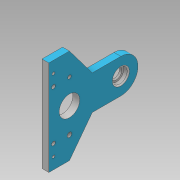
# Autodesk Inventor part: 탑(모터쪽옆면수정)
Saved by Autodesk Inventor 2018 (Build 220112000, 112)
## iProperties
Created: 2018-04-17
Part Number: 탑(모터쪽옆면수정)
Material: 일반
Document SubType Name: Modeling
Designer: CK
Density: 1 g/cm^3
Appearance: 기본값
Mass: 19.8797 g
Surface Area: 92.9275 cm^2
Volume: 19.8797 cm^3
Author: CK
Autodesk Inventor part; units mm, degrees
ref_plane "YZ Plane" through (0, 0, 0) normal (1, 0, 0) x (0, 1, 0)
ref_plane "XZ Plane" through (0, 0, 0) normal (0, 1, 0) x (-1, 0, 0)
ref_plane "XY Plane" through (0, 0, 0) normal (0, 0, 1) x (1, 0, 0)
sketch "스케치1" plane through (0, 0, 0) normal (1, 0, 0) x (0, 1, 0)
  line L0 (0, -41.5) -> (18, -41.5)
  line L1 (18, -41.5) -> (18, 59.6584) construction
  line L2 (0, 0) -> (0, -41.5)
  line L3 (84.3904, 0) -> (-15.1692, 0) construction
  arc A0 (63, -15) -> (78, 0) centre (63, 0) ccw
  line L4 (63, -15) -> (38, -15)
  line L5 (38, -15) -> (18, -41.5)
  line L6 (0, 41.5) -> (18, 41.5)
  line L7 (0, 0) -> (0, 41.5)
  arc A1 (78, 0) -> (63, 15) centre (63, 0) ccw
  line L8 (63, 15) -> (38, 15)
  line L9 (38, 15) -> (18, 41.5)
  dimension "d0" = 18
  dimension "d8" = 45
  dimension "d9" = 25
  constraints: 20 end point, 4 point on circle, 4 symmetric about line, 2 centre point, 2 horizontal, 2 point on line, 2 vertical, 1 other
  measures "d0" distance of L0.start L0.end
  measures "d8" distance from line of L1 A0.centre
  measures "d9" distance of L4.start L4.end
extrude "돌출1" add sketch "스케치1" along normal blind 6
sketch "스케치2" plane through (6, 0, 0) normal (1, 0, 0) x (0, 0, -1)
  line L0 (-58.8675, 4) -> (65.7315, 4) construction
  line L1 (-41.5, 0) -> (41.5, 0) projected
  circle A0 centre (31.5, 4) radius 1.15
  circle A1 centre (21.5, 4) radius 1.65
  line L2 (41.5, 0) -> (41.5, 18) projected
  line L3 (0, 13.8041) -> (0, -7.7982) construction
  circle A2 centre (-31.5, 4) radius 1.15
  circle A3 centre (-21.5, 4) radius 1.65
  point P0 (0, 0)
  dimension "d12" = 4
  dimension "d13" = 2.3
  dimension "d14" = 3.3
  dimension "d15" = 10
  dimension "d16" = 20
  dimension "d32" = 21.5
  constraints: 4 centre point, 4 end point, 2 point on line, 2 symmetric about line, 1 horizontal, 1 vertical, 2 other
  measures "d12" distance between parallel lines of L1 L0
  measures "d13" diameter of A0
  measures "d14" diameter of A1
  measures "d15" distance from line of L2 A0.centre
  measures "d16" distance from line of L2 A1.centre
  measures "d32" distance from line of L3 A1.centre
extrude "돌출2" cut sketch "스케치2" against normal blind 6
sketch "스케치3" plane through (6, 0, 0) normal (1, 0, 0) x (0, 0, -1)
  line L0 (-41.5, 18) -> (-41.5, 0) projected
  line L1 (41.5, 0) -> (41.5, 18) projected
  line L2 (-41.5, 18) -> (41.5, 18) construction
  line L3 (-21.915, 37.5775) -> (-21.915, 10.4705) construction
  line L4 (0, 43.7434) -> (0, -15.8221) construction
  line L5 (21.915, 37.5775) -> (21.915, 10.4705) construction
  circle A0 centre (-21.915, 18) radius 1.5
  circle A1 centre (21.915, 18) radius 2
  circle A2 centre (0, 18) radius 9
  point P0 (0, 0)
  dimension "d19" = 21.915
  dimension "d20" = 3
  dimension "d21" = 4
  dimension "d22" = 18
  constraints: 8 end point, 5 point on line, 3 centre point, 2 symmetric about line, 2 vertical, 1 horizontal, 1 midpoint
  measures "d19" distance from line of point (0, 0) L3
  measures "d20" diameter of A0
  measures "d21" diameter of A1
  measures "d22" diameter of A2
extrude "돌출3" cut sketch "스케치3" against normal blind 6
sketch "스케치4" plane through (6, 0, 0) normal (1, 0, 0) x (0, 0, -1)
  arc A0 (15, 63) -> (-15, 63) centre (0, 63) ccw projected
  circle A1 centre (0, 63) radius 6.5
  point P0 (0, 0)
  dimension "d25" = 13
  constraints: 1 centre point, 1 coincident
  measures "d25" diameter of A1
extrude "돌출4" cut sketch "스케치4" against normal blind 4
sketch "스케치5" plane through (2, 63, 0) normal (1, 0, 0) x (0, 0, -1)
  circle A0 centre (0, 0) radius 4.85
  point P0 (0, -63)
  dimension "d28" = 9.7
  constraints: 1 centre point
  measures "d28" diameter of A0
extrude "돌출5" cut sketch "스케치5" against normal blind 2
fillet "모깎기1" radius 1 1 edges at (6, 63, 6.5)
